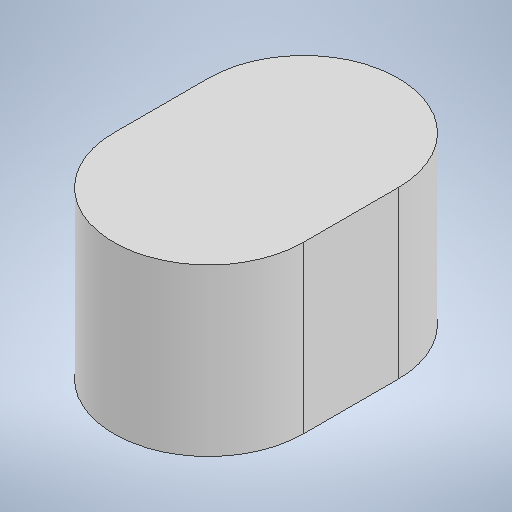
# Autodesk Inventor part: 45-01-002
Saved by Autodesk Inventor 2025.2 (Build 292293000, 293)
## iProperties
Created: 2024-11-28
Part Number: 45-01-002
Material: Generic
Document SubType Name: Modeling
Designer: Zvonko.Gabric
Density: 1 g/cm^3
Appearance: Default
Author: Zvonko.Gabric
Autodesk Inventor part; units mm, degrees
ref_plane "YZ Plane" through (0, 0, 0) normal (1, 0, 0) x (0, 1, 0)
ref_plane "XZ Plane" through (0, 0, 0) normal (0, 1, 0) x (-1, 0, 0)
ref_plane "XY Plane" through (0, 0, 0) normal (0, 0, 1) x (1, 0, 0)
sketch "Sketch1" plane through (0, 0, 0) normal (0, 1, 0) x (-1, 0, 0)
  line L0 (0, 0) -> (0, 4) construction
  line L1 (4, 0) -> (4, 4)
  line L2 (-4, 4) -> (-4, 0)
  arc A0 (-4, 0) -> (4, 0) centre (0, 0) ccw
  arc A1 (4, 4) -> (-4, 4) centre (0, 4) ccw
  point P0 (0, 2)
  dimension "d0" = 8
  dimension "d1" = 4
  constraints: 8 end point, 4 point on circle, 4 tangent, 2 centre point, 1 midpoint, 1 parallel, 1 vertical
  measures "d0" distance between parallel lines of L2 L1
  measures "d1" distance of L0.start L0.end
extrude "Extrusion1" add sketch "Sketch1" along normal blind 7
body "Solid1"
